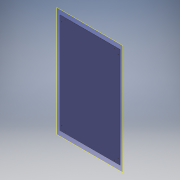
# Autodesk Inventor part: vrRig_v8_enclosure_topPanel
Saved by Autodesk Inventor 2016 (Build 200138000, 138)
## iProperties
Created: 2018-01-18
Part Number: vrRig_v8_enclosure_topPanel
Material: Generic
Document SubType Name: Modeling
Designer: harveylab
Density: 1 g/cm^3
Appearance: Default
Author: harveylab
Autodesk Inventor part; units mm, degrees
ref_plane "YZ Plane" through (0, 0, 0) normal (1, 0, 0) x (0, 1, 0)
ref_plane "XZ Plane" through (0, 0, 0) normal (0, 1, 0) x (-1, 0, 0)
ref_plane "XY Plane" through (0, 0, 0) normal (0, 0, 1) x (1, 0, 0)
ref_plane "Work Plane1" through (204.4192, -355.3778, -520.2745) normal (0, 0, -1) x (0, -1, 0)
sketch "Sketch1" plane through (204.4192, -355.3778, -520.2745) normal (0, 0, -1) x (0, -1, 0)
  line L0 (355.8032, 202.9143) -> (355.8032, -203.4857) projected
  line L1 (380.7, 225.6) -> (380.7, -225.6) projected
  line L2 (-378, 228.3) -> (378, 228.3) projected
  circle A0 centre (368.3, 190.5) radius 3.5 projected
  circle A1 centre (342.9, 215.9) radius 3.5 projected
  circle A2 centre (368.3, -190.5) radius 3.5 projected
  circle A3 centre (342.9, -215.9) radius 3.5 projected
  circle A4 centre (-342.9, -215.9) radius 3.5 projected
  circle A5 centre (-368.3, -190.5) radius 3.5 projected
  circle A6 centre (-368.3, 190.5) radius 3.5 projected
  circle A7 centre (-342.9, 215.9) radius 3.5 projected
  line L3 (380.7, 228.3) -> (-381.3, 228.3)
  line L4 (-381.3, 228.3) -> (-381.3, -228.9)
  line L5 (-381.3, -228.9) -> (380.7, -228.9)
  line L6 (380.7, -228.9) -> (380.7, 228.3)
  point P0 (-355.3778, 204.4192)
  dimension "d0" = 762
  dimension "d1" = 457.2
  constraints: 8 end point, 2 parallel, 1 horizontal, 1 perpendicular
  measures "d0" distance of L5.end L4.end
  measures "d1" distance of L4.end L3.end
extrude "Extrusion1" add sketch "Sketch1" along normal blind 1.5875
body "Solid1"
